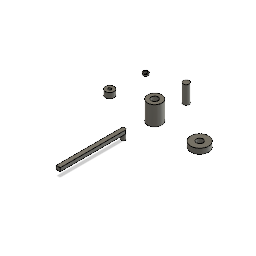
HotStuff v4 (Autodesk Fusion 360 design; units mm, degrees)
Autodesk Fusion 360 part; units mm, degrees
sketch "Sketch1" plane through (0, 0, 0) normal (0, 1, 0) x (1, 0, 0)
  circle A0 centre (0, 0) radius 3.7
  circle A1 centre (0, 0) radius 8
  dimension "d1" = 7.4
  dimension "d2" = 16
  constraint coincident A0.centre A1.centre
  constraint concentric A0 A1
  measures "d1" diameter of A0
  measures "d2" diameter of A1
extrude "Extrude1" add sketch "Sketch1" along normal blind 21.5 makes body 1
sketch "Sketch2" plane through (0, 0, 0) normal (0, 1, 0) x (1, 0, 0)
  circle A0 centre (-50, 0) radius 1.6
  circle A1 centre (-50, 0) radius 5
  dimension "d5" = 3.2
  dimension "d6" = 10
  constraint concentric A0 A1
  measures "d5" diameter of A0
  measures "d6" diameter of A1
extrude "Extrude2" add sketch "Sketch2" along normal blind 6 separate body makes body 2
sketch "Sketch3" plane through (0, 0, 0) normal (0, 1, 0) x (1, 0, 0)
  circle A0 centre (50, 0) radius 3.7
  circle A1 centre (50, 0) radius 10
  dimension "d9" = 7.4
  dimension "d10" = 20
  constraint concentric A0 A1
  measures "d9" diameter of A0
  measures "d10" diameter of A1
extrude "Extrude3" add sketch "Sketch3" along normal blind 6 separate body makes body 3
sketch "Sketch4" plane through (0, 0, 0) normal (0, 1, 0) x (1, 0, 0)
  circle A0 centre (0, 35) radius 3.45
  dimension "d13" = 6.9
  measures "d13" diameter of A0
extrude "Extrude4" add sketch "Sketch4" along normal blind 20 separate body makes body 4
sketch "Sketch5" plane through (0, 0, 0) normal (0, 1, 0) x (1, 0, 0)
  circle A0 centre (0, -35) radius 2.35
  dimension "d16" = 4.7
  measures "d16" diameter of A0
extrude "Extrude5" add sketch "Sketch5" along normal blind 6 separate body makes body 5
sketch "Sketch6" plane through (0, 6, 0) normal (0, 1, 0) x (-1, 0, 0)
  circle A0 centre (0, 35) radius 2.35
  circle A1 centre (0, 35) radius 2.35
  constraint concentric A0 A1
extrude "Extrude6" add sketch "Sketch6" along normal blind 4 bodies 5
ref_plane "WorkPlane1" through (0, 6.5991, 37.35) normal (0, 0, 1) x (-1, 0, 0)
sketch "Sketch7" plane through (0, 6.5991, 37.35) normal (0, 0, 1) x (1, 0, 0)
  line L0 (2.35, 3.4009) -> (-2.35, 3.4009)
  line L1 (2.35, -6.5991) -> (-2.35, -6.5991)
  line L2 (2.35, -6.5991) -> (2.35, 3.4009)
  line L3 (-2.35, -6.5991) -> (-2.35, 3.4009)
  line L4 (-2.35, 3.4009) -> (2.35, 3.4009)
  line L5 (2.35, 3.4009) -> (2.35, -0.5991)
  line L6 (2.35, -0.5991) -> (-2.35, -0.5991)
  line L7 (-2.35, -0.5991) -> (-2.35, 3.4009)
  dimension "d22" = 4
  constraint horizontal L4
  constraint vertical L5
  constraint horizontal L6
  constraint vertical L7
  constraint coincident L0.end L3.end
  measures "d22" distance of L0.end L6.end
extrude "Extrude7" add sketch "Sketch7" along normal blind 70 separate body contours L0 L2 L3 L4 L5 L6 L7 makes body 6
extrude "Extrude8" add 1 faces at (-0.7833, 8.6667, 37.35) along direction (0, 0, -1) blind 2.5 on bodies 6 bodies 6 5
sketch "Sketch8" plane through (0, 0, 0) normal (0, 1, 0) x (1, 0, 0)
  circle A0 centre (-50, 40) radius 1.75
  circle A1 centre (-50, 40) radius 3
  dimension "d27" = 3.5
  dimension "d28" = 6
  constraint concentric A0 A1
  measures "d27" diameter of A0
  measures "d28" diameter of A1
extrude "Extrude9" add sketch "Sketch8" along normal blind 2 separate body makes body 7
